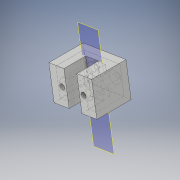
# Autodesk Inventor part: wrench holder
Saved by Autodesk Inventor 2017 (Build 210142000, 142)
## iProperties
Created: 2017-02-16
Part Number: wrench holder
Material: Generic
Document SubType Name: Modeling
Designer: kingb
Density: 1 g/cm^3
Appearance: Default
Author: kingb
Autodesk Inventor part; units mm, degrees
ref_plane "YZ Plane" through (0, 0, 0) normal (1, 0, 0) x (0, 1, 0)
ref_plane "XZ Plane" through (0, 0, 0) normal (0, 1, 0) x (-1, 0, 0)
ref_plane "Work Plane1" through (1.0078, -6.2592, 14.7955) normal (0, 0, -1) x (0.9872698, 0.1590547, 0)
sketch "Sketch1" plane through (1.0078, -6.2592, 14.7955) normal (0, 0, -1) x (0.9872698, 0.1590547, 0)
  circle A0 centre (12.6864, -4.6373) radius 2.9337 projected
  circle A1 centre (-12.7136, -4.6337) radius 2.9337 projected
  line L0 (25.2845, 14.4163) -> (-25.5155, 14.4163)
  line L1 (-25.5155, 14.4163) -> (-25.5155, -23.6837)
  line L2 (-25.5155, -23.6837) -> (25.2845, -23.6837)
  line L3 (25.2845, -23.6837) -> (25.2845, 14.4163)
  point P0 (0.0006, -6.3398)
  dimension "d0" = 50.8
  dimension "d1" = 38.1
  dimension "d2" = 19.05
  dimension "d3" = 12.8018
  constraints: 8 end point, 2 parallel, 1 horizontal, 1 perpendicular
  measures "d0" distance of L2.end L1.end
  measures "d1" distance between parallel lines of L2 L0
  measures "d2" distance from line of A1.centre L0
  measures "d3" distance from line of A1.centre L1
ref_plane "Work Plane2" through (-93.6315, -146.1207, 0) normal (0, 0, 1) x (1, 0, 0)
extrude "Extrusion1" add sketch "Sketch1" along normal up to surface (14.7955 mm away)
sketch "Sketch2" plane through (1.0078, -6.2592, 14.7955) normal (0, 0, 1) x (0.9872698, 0.1590547, 0)
  line L0 (6.35, -58.321) -> (6.35, 48.9196) projected
  line L1 (-6.35, 49.2476) -> (-6.35, -58.321) projected
  circle A0 centre (-12.7136, 4.6337) radius 2.9337 projected
  circle A1 centre (12.6864, 4.6373) radius 2.9337 projected
  line L2 (25.2845, -14.4163) -> (-25.5155, -14.4163) projected
  line L3 (25.2845, 23.6837) -> (25.2845, -14.4163) projected
  line L4 (-25.5155, 23.6837) -> (25.2845, 23.6837) projected
  line L5 (-25.5155, -14.4163) -> (-25.5155, 23.6837) projected
  line L6 (25.2845, -14.4163) -> (-25.5155, -14.4163) projected
  line L7 (25.2845, -14.4163) -> (7.62, -14.4163)
  line L8 (7.62, -14.4163) -> (7.62, 23.6837)
  line L9 (7.62, 23.6837) -> (25.2845, 23.6837)
  line L10 (25.2845, 23.6837) -> (25.2845, -14.4163)
  line L11 (-25.5155, -14.4163) -> (-25.5155, 23.6837) projected
  line L12 (-25.5155, -14.4163) -> (-7.62, -14.4163)
  line L13 (-7.62, -14.4163) -> (-7.62, 23.6837)
  line L14 (-7.62, 23.6837) -> (-25.5155, 23.6837)
  line L15 (-25.5155, 23.6837) -> (-25.5155, -14.4163)
  point P0 (0.0006, 6.3398)
  dimension "d6" = 1.27
  dimension "d7" = 1.27
  constraints: 16 end point, 4 parallel, 2 horizontal, 2 perpendicular, 2 point on line
  measures "d6" distance between parallel lines of L1 L13
  measures "d7" distance between parallel lines of L0 L8
extrude "Extrusion2" add sketch "Sketch2" along normal blind 25.4 contours L8 L4 L3 L2 | L2 L5 L4 L13
shell "Shell1" thickness 3.81 removed faces 0
body "Solid1"
